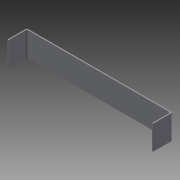
# Autodesk Inventor part: Conveyor Brace
Saved by Autodesk Inventor 2015 (Build 190159000, 159)
## iProperties
Created: 2015-01-26
Part Number: Conveyor Brace
Material: Generic
Document SubType Name: Modeling
Designer: chapale16
Density: 1 g/cm^3
Appearance: Default
Author: chapale16
Autodesk Inventor part; units mm, degrees
ref_plane "YZ Plane" through (0, 0, 0) normal (1, 0, 0) x (0, 1, 0)
ref_plane "XZ Plane" through (0, 0, 0) normal (0, 1, 0) x (-1, 0, 0)
ref_plane "XY Plane" through (0, 0, 0) normal (0, 0, 1) x (1, 0, 0)
sketch "Sketch1" plane through (0, 0, 0) normal (0, 0, 1) x (1, 0, 0)
  line L0 (0, 0) -> (304.8, 0)
  line L1 (304.8, 0) -> (304.8, -50.8)
  line L2 (304.8, -50.8) -> (0, -50.8)
  line L3 (0, -50.8) -> (0, 0)
  dimension "d0" = 304.8
  dimension "d1" = 50.8
  constraints: 8 end point, 2 parallel, 1 horizontal, 1 perpendicular
  measures "d0" distance of L1.end L2.end
  measures "d1" distance of L0.end L1.end
extrude "Extrusion1" add sketch "Sketch1" along normal blind 2.2098
sketch "Sketch2" plane through (0, 0, 2.2098) normal (0, 0, 1) x (1, 0, 0)
  line L0 (0, -50.8) -> (304.8, -50.8) projected
  line L1 (0, 0) -> (2.2098, 0)
  line L2 (2.2098, 0) -> (2.2098, -50.8)
  line L3 (2.2098, -50.8) -> (0, -50.8)
  line L4 (0, -50.8) -> (0, 0)
  line L5 (304.8, 0) -> (302.5902, 0)
  line L6 (302.5902, 0) -> (302.5902, -50.8)
  line L7 (302.5902, -50.8) -> (304.8, -50.8)
  line L8 (304.8, -50.8) -> (304.8, 0)
  dimension "d4" = 2.2098
  dimension "d5" = 2.2098
  constraints: 16 end point, 4 parallel, 3 point on line, 2 horizontal, 2 perpendicular
  measures "d4" distance of L2.end L3.end
  measures "d5" distance of L7.end L6.end
extrude "Extrusion2" add sketch "Sketch2" along normal blind 50.8
fillet "Fillet1" radius 3.175 1 edges at (304.8, -25.4, 0)
fillet "Fillet2" radius 3.175 1 edges at (0, -25.4, 0)
fillet "Fillet3" radius 3.175 1 edges at (2.2098, -25.4, 2.2098)
fillet "Fillet4" radius 3.175 1 edges at (302.5902, -25.4, 2.2098)
sketch "Sketch3" plane through (304.8, -50.8, 53.0098) normal (1, 0, 0) x (0, 0, -1)
  line L0 (0, 0) -> (12.3698, 0)
  line L1 (49.8348, 0) -> (0, 0) projected
  line L2 (12.3698, 0) -> (12.3698, 65.8948)
  line L3 (47.625, 50.8) -> (0, 50.8) projected
  line L4 (12.3698, 65.8948) -> (-20.1931, 65.8948)
  line L5 (-20.1931, 65.8948) -> (-20.1931, 0)
  line L6 (-20.1931, 0) -> (12.3698, 0)
  point P0 (53.0098, 50.8)
  dimension "d12" = 12.3698
  constraints: 10 end point, 3 perpendicular, 2 point on line, 1 collinear
  measures "d12" distance of L0.start L0.end
extrude "Extrusion3" cut sketch "Sketch3" against normal through all
body "Solid1"
